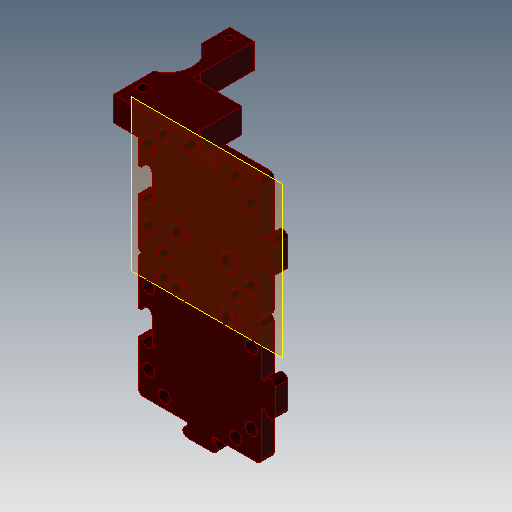
# Autodesk Inventor part: 30_cellSTORM_base
Saved by Autodesk Inventor 2019.4 (Build 234330000, 330)
## iProperties
Created: 2021-07-06
Part Number: 30_cellSTORM_base
Material: Generic
Document SubType Name: Modeling
Designer: diederichbenedict
Density: 1 g/cm^3
Appearance: Smooth - Red
Mass: 29.7217 g
Surface Area: 152.077 cm^2
Volume: 29.7217 cm^3
Author: diederichbenedict
Autodesk Inventor part; units mm, degrees
ref_plane "YZ Plane" through (0, 0, 0) normal (1, 0, 0) x (0, 1, 0)
ref_plane "XZ Plane" through (0, 0, 0) normal (0, 1, 0) x (-1, 0, 0)
ref_plane "XY Plane" through (0, 0, 0) normal (0, 0, 1) x (1, 0, 0)
ref_plane "Work Plane1" through (0, 0, 0) normal (0, 0, 1) x (1, 0, 0)
sketch "Sketch1" plane through (0, 0, 0) normal (0, 0, 1) x (1, 0, 0)
  circle A0 centre (5.7948, 15.4052) radius 2.5 construction
  circle A1 centre (-15.6052, -5.7948) radius 2.5 construction
  line L0 (-20.0856, 39.0762) -> (-20.0856, 40.2052) construction
  line L1 (-20.0856, 40.2052) -> (-38.2052, 40.2052) construction
  arc A2 (-38.2052, 40.2052) -> (-40.2052, 38.2052) centre (-38.2052, 38.2052) ccw construction
  line L2 (-40.2052, 20.2953) -> (-40.2052, 38.2052) construction
  line L3 (-40.2052, 20.2953) -> (-39.0783, 20.2953) construction
  arc A3 (-39.0783, 20.2953) -> (-38.6768, 20.6232) centre (-39.0783, 20.7051) ccw construction
  arc A4 (-34.5391, 20.2052) -> (-38.6768, 20.6232) centre (-36.6291, 20.2052) ccw construction
  line L4 (-34.5391, 20.2052) -> (-34.5391, 10.4067) construction
  arc A5 (-38.647, 9.8643) -> (-34.5391, 10.4067) centre (-36.6023, 10.2052) ccw construction
  line L5 (-38.647, 9.8643) -> (-38.6775, 9.9849) construction
  arc A6 (-38.6775, 9.9849) -> (-39.0762, 10.3249) centre (-39.083, 9.9131) ccw construction
  line L6 (-39.0762, 10.3249) -> (-40.2052, 10.3249) construction
  line L7 (-40.2052, -7.7948) -> (-40.2052, 10.3249) construction
  arc A7 (-40.2052, -7.7948) -> (-38.2052, -9.7948) centre (-38.2052, -7.7948) ccw construction
  line L8 (-38.2052, -9.7948) -> (-20.2052, -9.7948) construction
  line L9 (-20.2052, -9.7948) -> (-20.2052, -10.8453) construction
  arc A8 (-20.6052, -11.3352) -> (-20.2052, -10.8453) centre (-20.7052, -10.8453) ccw construction
  arc A9 (-20.6052, -11.3352) -> (-20.2052, -15.2948) centre (-20.2052, -13.2948) ccw construction
  line L10 (-20.2052, -15.2948) -> (-10.2052, -15.2948) construction
  arc A10 (-10.2052, -15.2948) -> (-9.8052, -11.3352) centre (-10.2052, -13.2948) ccw construction
  arc A11 (-10.2052, -10.8453) -> (-9.8052, -11.3352) centre (-9.7052, -10.8453) ccw construction
  line L11 (-10.2052, -10.8453) -> (-10.2052, -9.7948) construction
  line L12 (-10.2052, -9.7948) -> (7.7948, -9.7948) construction
  arc A12 (7.7948, -9.7948) -> (9.7948, -7.7948) centre (7.7948, -7.7948) ccw construction
  line L13 (9.7948, 10.2052) -> (9.7948, -7.7948) construction
  line L14 (9.7948, 10.2052) -> (10.8453, 10.2052) construction
  arc A13 (11.3352, 9.8052) -> (10.8453, 10.2052) centre (10.8453, 9.7052) ccw construction
  arc A14 (11.3352, 9.8052) -> (15.2948, 10.2052) centre (13.2948, 10.2052) ccw construction
  line L15 (15.2948, 10.2052) -> (15.2948, 20.2052) construction
  arc A15 (15.2948, 20.2052) -> (11.3352, 20.6052) centre (13.2948, 20.2052) ccw construction
  arc A16 (10.8453, 20.2052) -> (11.3352, 20.6052) centre (10.8453, 20.7052) ccw construction
  line L16 (10.8453, 20.2052) -> (9.7948, 20.2052) construction
  line L17 (9.7948, 38.2052) -> (9.7948, 20.2052) construction
  arc A17 (9.7948, 38.2052) -> (7.7948, 40.2052) centre (7.7948, 38.2052) ccw construction
  line L18 (7.7948, 40.2052) -> (-10.1151, 40.2052) construction
  line L19 (-10.1151, 40.2052) -> (-10.1151, 39.0783) construction
  arc A18 (-10.1151, 39.0783) -> (-9.7873, 38.6768) centre (-9.7054, 39.0783) ccw construction
  arc A19 (-10.2052, 34.5391) -> (-9.7873, 38.6768) centre (-10.2052, 36.6291) ccw construction
  line L20 (-10.2052, 34.5391) -> (-20.0038, 34.5391) construction
  arc A20 (-20.5462, 38.647) -> (-20.0038, 34.5391) centre (-20.2052, 36.6023) ccw construction
  line L21 (-20.5462, 38.647) -> (-20.4256, 38.6775) construction
  arc A21 (-20.4256, 38.6775) -> (-20.0856, 39.0762) centre (-20.4974, 39.083) ccw construction
  line L22 (-0.2052, 32.2052) -> (-30.2052, 32.2052) construction
  arc A22 (1.7948, 30.2052) -> (-0.2052, 32.2052) centre (-0.2052, 30.2052) ccw construction
  line L23 (1.7948, 30.2052) -> (1.7948, 0.2052) construction
  arc A23 (-0.2052, -1.7948) -> (1.7948, 0.2052) centre (-0.2052, 0.2052) ccw construction
  line L24 (-0.2052, -1.7948) -> (-30.2052, -1.7948) construction
  arc A24 (-32.2052, 0.2052) -> (-30.2052, -1.7948) centre (-30.2052, 0.2052) ccw construction
  line L25 (-32.2052, 0.2052) -> (-32.2052, 30.2052) construction
  arc A25 (-30.2052, 32.2052) -> (-32.2052, 30.2052) centre (-30.2052, 30.2052) ccw construction
  circle A26 centre (-35.2052, 35.2052) radius 2.425 construction
  circle A27 centre (-29.7052, 36.0052) radius 2.65 construction
  circle A28 centre (-36.0052, 29.7052) radius 2.65 construction
  circle A29 centre (-35.2052, -4.7948) radius 2.425 construction
  circle A30 centre (-29.7052, -5.5948) radius 2.65 construction
  circle A31 centre (-36.0052, 0.7052) radius 2.65 construction
  circle A32 centre (4.7948, 35.2052) radius 2.425 construction
  circle A33 centre (-0.7052, 36.0052) radius 2.65 construction
  circle A34 centre (5.5948, 29.7052) radius 2.65 construction
  circle A35 centre (5.5948, 0.7052) radius 2.65 construction
  circle A36 centre (-0.7052, -5.5948) radius 2.65 construction
  circle A37 centre (4.7948, -4.7948) radius 2.425 construction
  circle A38 centre (5.7948, -34.5948) radius 2.5 construction
  circle A39 centre (-15.6052, -55.7948) radius 2.5 construction
  line L26 (-20.0856, -10.9238) -> (-20.0856, -9.7948) construction
  line L27 (-20.0856, -9.7948) -> (-38.2052, -9.7948) construction
  arc A40 (-38.2052, -9.7948) -> (-40.2052, -11.7948) centre (-38.2052, -11.7948) ccw construction
  line L28 (-40.2052, -29.7047) -> (-40.2052, -11.7948) construction
  line L29 (-40.2052, -29.7047) -> (-39.0783, -29.7047) construction
  arc A41 (-39.0783, -29.7047) -> (-38.6768, -29.3768) centre (-39.0783, -29.2949) ccw construction
  arc A42 (-34.5391, -29.7948) -> (-38.6768, -29.3768) centre (-36.6291, -29.7948) ccw construction
  line L30 (-34.5391, -29.7948) -> (-34.5391, -39.5933) construction
  arc A43 (-38.647, -40.1357) -> (-34.5391, -39.5933) centre (-36.6023, -39.7948) ccw construction
  line L31 (-38.647, -40.1357) -> (-38.6775, -40.0151) construction
  arc A44 (-38.6775, -40.0151) -> (-39.0762, -39.6751) centre (-39.083, -40.0869) ccw construction
  line L32 (-39.0762, -39.6751) -> (-40.2052, -39.6751) construction
  line L33 (-40.2052, -57.7948) -> (-40.2052, -39.6751) construction
  arc A45 (-40.2052, -57.7948) -> (-38.2052, -59.7948) centre (-38.2052, -57.7948) ccw construction
  line L34 (-38.2052, -59.7948) -> (-20.2052, -59.7948) construction
  line L35 (-20.2052, -59.7948) -> (-20.2052, -60.8453) construction
  arc A46 (-20.6052, -61.3352) -> (-20.2052, -60.8453) centre (-20.7052, -60.8453) ccw construction
  arc A47 (-20.6052, -61.3352) -> (-20.2052, -65.2948) centre (-20.2052, -63.2948) ccw construction
  line L36 (-20.2052, -65.2948) -> (-10.2052, -65.2948) construction
  arc A48 (-10.2052, -65.2948) -> (-9.8052, -61.3352) centre (-10.2052, -63.2948) ccw construction
  arc A49 (-10.2052, -60.8453) -> (-9.8052, -61.3352) centre (-9.7052, -60.8453) ccw construction
  line L37 (-10.2052, -60.8453) -> (-10.2052, -59.7948) construction
  line L38 (-10.2052, -59.7948) -> (7.7948, -59.7948) construction
  arc A50 (7.7948, -59.7948) -> (9.7948, -57.7948) centre (7.7948, -57.7948) ccw construction
  line L39 (9.7948, -39.7948) -> (9.7948, -57.7948) construction
  line L40 (9.7948, -39.7948) -> (10.8453, -39.7948) construction
  arc A51 (11.3352, -40.1948) -> (10.8453, -39.7948) centre (10.8453, -40.2948) ccw construction
  arc A52 (11.3352, -40.1948) -> (15.2948, -39.7948) centre (13.2948, -39.7948) ccw construction
  line L41 (15.2948, -39.7948) -> (15.2948, -29.7948) construction
  arc A53 (15.2948, -29.7948) -> (11.3352, -29.3948) centre (13.2948, -29.7948) ccw construction
  arc A54 (10.8453, -29.7948) -> (11.3352, -29.3948) centre (10.8453, -29.2948) ccw construction
  line L42 (10.8453, -29.7948) -> (9.7948, -29.7948) construction
  line L43 (9.7948, -11.7948) -> (9.7948, -29.7948) construction
  arc A55 (9.7948, -11.7948) -> (7.7948, -9.7948) centre (7.7948, -11.7948) ccw construction
  line L44 (7.7948, -9.7948) -> (-10.1151, -9.7948) construction
  line L45 (-10.1151, -9.7948) -> (-10.1151, -10.9217) construction
  arc A56 (-10.1151, -10.9217) -> (-9.7873, -11.3232) centre (-9.7054, -10.9217) ccw construction
  arc A57 (-10.2052, -15.4609) -> (-9.7873, -11.3232) centre (-10.2052, -13.3709) ccw construction
  line L46 (-10.2052, -15.4609) -> (-20.0038, -15.4609) construction
  arc A58 (-20.5462, -11.353) -> (-20.0038, -15.4609) centre (-20.2052, -13.3977) ccw construction
  line L47 (-20.5462, -11.353) -> (-20.4256, -11.3225) construction
  arc A59 (-20.4256, -11.3225) -> (-20.0856, -10.9238) centre (-20.4974, -10.917) ccw construction
  line L48 (-0.2052, -17.7948) -> (-30.2052, -17.7948) construction
  arc A60 (1.7948, -19.7948) -> (-0.2052, -17.7948) centre (-0.2052, -19.7948) ccw construction
  line L49 (1.7948, -19.7948) -> (1.7948, -49.7948) construction
  arc A61 (-0.2052, -51.7948) -> (1.7948, -49.7948) centre (-0.2052, -49.7948) ccw construction
  line L50 (-0.2052, -51.7948) -> (-30.2052, -51.7948) construction
  arc A62 (-32.2052, -49.7948) -> (-30.2052, -51.7948) centre (-30.2052, -49.7948) ccw construction
  line L51 (-32.2052, -49.7948) -> (-32.2052, -19.7948) construction
  arc A63 (-30.2052, -17.7948) -> (-32.2052, -19.7948) centre (-30.2052, -19.7948) ccw construction
  circle A64 centre (-35.2052, -14.7948) radius 2.425 construction
  circle A65 centre (-29.7052, -13.9948) radius 2.65 construction
  circle A66 centre (-36.0052, -20.2948) radius 2.65 construction
  circle A67 centre (-35.2052, -54.7948) radius 2.425 construction
  circle A68 centre (-29.7052, -55.5948) radius 2.65 construction
  circle A69 centre (-36.0052, -49.2948) radius 2.65 construction
  circle A70 centre (4.7948, -14.7948) radius 2.425 construction
  circle A71 centre (-0.7052, -13.9948) radius 2.65 construction
  circle A72 centre (5.5948, -20.2948) radius 2.65 construction
  circle A73 centre (5.5948, -49.2948) radius 2.65 construction
  circle A74 centre (-0.7052, -55.5948) radius 2.65 construction
  circle A75 centre (4.7948, -54.7948) radius 2.425 construction
  circle A76 centre (5.7948, 15.4052) radius 2.5 projected
  circle A77 centre (-15.6052, -5.7948) radius 2.5 projected
  line L52 (-20.0856, 39.0762) -> (-20.0856, 40.2052) projected
  line L53 (-20.0856, 40.2052) -> (-38.2052, 40.2052) projected
  arc A78 (-38.2052, 40.2052) -> (-40.2052, 38.2052) centre (-38.2052, 38.2052) ccw projected
  line L54 (-40.2052, 20.2953) -> (-40.2052, 38.2052) projected
  line L55 (-40.2052, 20.2953) -> (-39.0783, 20.2953) projected
  arc A79 (-39.0783, 20.2953) -> (-38.6768, 20.6232) centre (-39.0783, 20.7051) ccw projected
  arc A80 (-34.5391, 20.2052) -> (-38.6768, 20.6232) centre (-36.6291, 20.2052) ccw projected
  line L56 (-34.5391, 20.2052) -> (-34.5391, 10.4067) projected
  arc A81 (-38.647, 9.8643) -> (-34.5391, 10.4067) centre (-36.6023, 10.2052) ccw projected
  line L57 (-38.647, 9.8643) -> (-38.6775, 9.9849) projected
  arc A82 (-38.6775, 9.9849) -> (-39.0762, 10.3249) centre (-39.083, 9.9131) ccw projected
  line L58 (-39.0762, 10.3249) -> (-40.2052, 10.3249) projected
  line L59 (-40.2052, -7.7948) -> (-40.2052, 10.3249) projected
  arc A83 (-40.2052, -7.7948) -> (-38.2052, -9.7948) centre (-38.2052, -7.7948) ccw projected
  line L60 (-38.2052, -9.7948) -> (-20.2052, -9.7948) projected
  line L61 (-20.2052, -9.7948) -> (-20.2052, -10.8453) projected
  arc A84 (-20.6052, -11.3352) -> (-20.2052, -10.8453) centre (-20.7052, -10.8453) ccw projected
  arc A85 (-20.6052, -11.3352) -> (-20.2052, -15.2948) centre (-20.2052, -13.2948) ccw projected
  line L62 (-20.2052, -15.2948) -> (-10.2052, -15.2948) projected
  arc A86 (-10.2052, -15.2948) -> (-9.8052, -11.3352) centre (-10.2052, -13.2948) ccw projected
  arc A87 (-10.2052, -10.8453) -> (-9.8052, -11.3352) centre (-9.7052, -10.8453) ccw projected
  line L63 (-10.2052, -10.8453) -> (-10.2052, -9.7948) projected
  line L64 (-10.2052, -9.7948) -> (7.7948, -9.7948) projected
  arc A88 (7.7948, -9.7948) -> (9.7948, -7.7948) centre (7.7948, -7.7948) ccw projected
  line L65 (9.7948, 10.2052) -> (9.7948, -7.7948) projected
  line L66 (9.7948, 10.2052) -> (10.8453, 10.2052) projected
  arc A89 (11.3352, 9.8052) -> (10.8453, 10.2052) centre (10.8453, 9.7052) ccw projected
  arc A90 (11.3352, 9.8052) -> (15.2948, 10.2052) centre (13.2948, 10.2052) ccw projected
  line L67 (15.2948, 10.2052) -> (15.2948, 20.2052) projected
  arc A91 (15.2948, 20.2052) -> (11.3352, 20.6052) centre (13.2948, 20.2052) ccw projected
  arc A92 (10.8453, 20.2052) -> (11.3352, 20.6052) centre (10.8453, 20.7052) ccw projected
  line L68 (10.8453, 20.2052) -> (9.7948, 20.2052) projected
  line L69 (9.7948, 38.2052) -> (9.7948, 20.2052) projected
  arc A93 (9.7948, 38.2052) -> (7.7948, 40.2052) centre (7.7948, 38.2052) ccw projected
  line L70 (7.7948, 40.2052) -> (-10.1151, 40.2052) projected
  line L71 (-10.1151, 40.2052) -> (-10.1151, 39.0783) projected
  arc A94 (-10.1151, 39.0783) -> (-9.7873, 38.6768) centre (-9.7054, 39.0783) ccw projected
  arc A95 (-10.2052, 34.5391) -> (-9.7873, 38.6768) centre (-10.2052, 36.6291) ccw projected
  line L72 (-10.2052, 34.5391) -> (-20.0038, 34.5391) projected
  arc A96 (-20.5462, 38.647) -> (-20.0038, 34.5391) centre (-20.2052, 36.6023) ccw projected
  line L73 (-20.5462, 38.647) -> (-20.4256, 38.6775) projected
  arc A97 (-20.4256, 38.6775) -> (-20.0856, 39.0762) centre (-20.4974, 39.083) ccw projected
  line L74 (-0.2052, 32.2052) -> (-30.2052, 32.2052) projected
  arc A98 (1.7948, 30.2052) -> (-0.2052, 32.2052) centre (-0.2052, 30.2052) ccw projected
  line L75 (1.7948, 30.2052) -> (1.7948, 0.2052) projected
  arc A99 (-0.2052, -1.7948) -> (1.7948, 0.2052) centre (-0.2052, 0.2052) ccw projected
  line L76 (-0.2052, -1.7948) -> (-30.2052, -1.7948) projected
  arc A100 (-32.2052, 0.2052) -> (-30.2052, -1.7948) centre (-30.2052, 0.2052) ccw projected
  line L77 (-32.2052, 0.2052) -> (-32.2052, 30.2052) projected
  arc A101 (-30.2052, 32.2052) -> (-32.2052, 30.2052) centre (-30.2052, 30.2052) ccw projected
  circle A102 centre (-35.2052, 35.2052) radius 2.425 projected
  circle A103 centre (-29.7052, 36.0052) radius 2.65 projected
  circle A104 centre (-36.0052, 29.7052) radius 2.65 projected
  circle A105 centre (-35.2052, -4.7948) radius 2.425 projected
  circle A106 centre (-29.7052, -5.5948) radius 2.65 projected
  circle A107 centre (-36.0052, 0.7052) radius 2.65 projected
  circle A108 centre (4.7948, 35.2052) radius 2.425 projected
  circle A109 centre (-0.7052, 36.0052) radius 2.65 projected
  circle A110 centre (5.5948, 29.7052) radius 2.65 projected
  circle A111 centre (5.5948, 0.7052) radius 2.65 projected
  circle A112 centre (-0.7052, -5.5948) radius 2.65 projected
  circle A113 centre (4.7948, -4.7948) radius 2.425 projected
  circle A114 centre (5.7948, -34.5948) radius 2.5 projected
  circle A115 centre (-15.6052, -55.7948) radius 2.5 projected
  line L78 (-20.0856, -10.9238) -> (-20.0856, -9.7948) projected
  line L79 (-20.0856, -9.7948) -> (-38.2052, -9.7948) projected
  arc A116 (-38.2052, -9.7948) -> (-40.2052, -11.7948) centre (-38.2052, -11.7948) ccw projected
  line L80 (-40.2052, -29.7047) -> (-40.2052, -11.7948) projected
  line L81 (-40.2052, -29.7047) -> (-39.0783, -29.7047) projected
  arc A117 (-39.0783, -29.7047) -> (-38.6768, -29.3768) centre (-39.0783, -29.2949) ccw projected
  arc A118 (-34.5391, -29.7948) -> (-38.6768, -29.3768) centre (-36.6291, -29.7948) ccw projected
  line L82 (-34.5391, -29.7948) -> (-34.5391, -39.5933) projected
  arc A119 (-38.647, -40.1357) -> (-34.5391, -39.5933) centre (-36.6023, -39.7948) ccw projected
  line L83 (-38.647, -40.1357) -> (-38.6775, -40.0151) projected
  arc A120 (-38.6775, -40.0151) -> (-39.0762, -39.6751) centre (-39.083, -40.0869) ccw projected
  line L84 (-39.0762, -39.6751) -> (-40.2052, -39.6751) projected
  line L85 (-40.2052, -57.7948) -> (-40.2052, -39.6751) projected
  arc A121 (-40.2052, -57.7948) -> (-38.2052, -59.7948) centre (-38.2052, -57.7948) ccw projected
  line L86 (-38.2052, -59.7948) -> (-20.2052, -59.7948) projected
  line L87 (-20.2052, -59.7948) -> (-20.2052, -60.8453) projected
  arc A122 (-20.6052, -61.3352) -> (-20.2052, -60.8453) centre (-20.7052, -60.8453) ccw projected
  arc A123 (-20.6052, -61.3352) -> (-20.2052, -65.2948) centre (-20.2052, -63.2948) ccw projected
  line L88 (-20.2052, -65.2948) -> (-10.2052, -65.2948) projected
  arc A124 (-10.2052, -65.2948) -> (-9.8052, -61.3352) centre (-10.2052, -63.2948) ccw projected
  arc A125 (-10.2052, -60.8453) -> (-9.8052, -61.3352) centre (-9.7052, -60.8453) ccw projected
  line L89 (-10.2052, -60.8453) -> (-10.2052, -59.7948) projected
  line L90 (-10.2052, -59.7948) -> (7.7948, -59.7948) projected
  arc A126 (7.7948, -59.7948) -> (9.7948, -57.7948) centre (7.7948, -57.7948) ccw projected
  line L91 (9.7948, -39.7948) -> (9.7948, -57.7948) projected
  line L92 (9.7948, -39.7948) -> (10.8453, -39.7948) projected
  arc A127 (11.3352, -40.1948) -> (10.8453, -39.7948) centre (10.8453, -40.2948) ccw projected
  arc A128 (11.3352, -40.1948) -> (15.2948, -39.7948) centre (13.2948, -39.7948) ccw projected
  line L93 (15.2948, -39.7948) -> (15.2948, -29.7948) projected
  arc A129 (15.2948, -29.7948) -> (11.3352, -29.3948) centre (13.2948, -29.7948) ccw projected
  arc A130 (10.8453, -29.7948) -> (11.3352, -29.3948) centre (10.8453, -29.2948) ccw projected
  line L94 (10.8453, -29.7948) -> (9.7948, -29.7948) projected
  line L95 (9.7948, -11.7948) -> (9.7948, -29.7948) projected
  arc A131 (9.7948, -11.7948) -> (7.7948, -9.7948) centre (7.7948, -11.7948) ccw projected
  line L96 (7.7948, -9.7948) -> (-10.1151, -9.7948) projected
  line L97 (-10.1151, -9.7948) -> (-10.1151, -10.9217) projected
  arc A132 (-10.1151, -10.9217) -> (-9.7873, -11.3232) centre (-9.7054, -10.9217) ccw projected
  arc A133 (-10.2052, -15.4609) -> (-9.7873, -11.3232) centre (-10.2052, -13.3709) ccw projected
  line L98 (-10.2052, -15.4609) -> (-20.0038, -15.4609) projected
  arc A134 (-20.5462, -11.353) -> (-20.0038, -15.4609) centre (-20.2052, -13.3977) ccw projected
  line L99 (-20.5462, -11.353) -> (-20.4256, -11.3225) projected
  arc A135 (-20.4256, -11.3225) -> (-20.0856, -10.9238) centre (-20.4974, -10.917) ccw projected
  line L100 (-0.2052, -17.7948) -> (-30.2052, -17.7948) projected
  arc A136 (1.7948, -19.7948) -> (-0.2052, -17.7948) centre (-0.2052, -19.7948) ccw projected
  line L101 (1.7948, -19.7948) -> (1.7948, -49.7948) projected
  arc A137 (-0.2052, -51.7948) -> (1.7948, -49.7948) centre (-0.2052, -49.7948) ccw projected
  line L102 (-0.2052, -51.7948) -> (-30.2052, -51.7948) projected
  arc A138 (-32.2052, -49.7948) -> (-30.2052, -51.7948) centre (-30.2052, -49.7948) ccw projected
  line L103 (-32.2052, -49.7948) -> (-32.2052, -19.7948) projected
  arc A139 (-30.2052, -17.7948) -> (-32.2052, -19.7948) centre (-30.2052, -19.7948) ccw projected
  circle A140 centre (-35.2052, -14.7948) radius 2.425 projected
  circle A141 centre (-29.7052, -13.9948) radius 2.65 projected
  circle A142 centre (-36.0052, -20.2948) radius 2.65 projected
  circle A143 centre (-35.2052, -54.7948) radius 2.425 projected
  circle A144 centre (-29.7052, -55.5948) radius 2.65 projected
  circle A145 centre (-36.0052, -49.2948) radius 2.65 projected
  circle A146 centre (4.7948, -14.7948) radius 2.425 projected
  circle A147 centre (-0.7052, -13.9948) radius 2.65 projected
  circle A148 centre (5.5948, -20.2948) radius 2.65 projected
  circle A149 centre (5.5948, -49.2948) radius 2.65 projected
  circle A150 centre (-0.7052, -55.5948) radius 2.65 projected
  circle A151 centre (4.7948, -54.7948) radius 2.425 projected
  point P0 (0, 0)
extrude "Extrusion1" add sketch "Sketch1" against normal blind 5 contours A76 | A77 | A97 L73 A96 L72 A95 A94 L71 L70 A93 L69 L68 A92 A91 L67 A90 A89 L66 L65 A88 L64 L63 A87 A86 L62 A85 A134 L99 A135 L78 L79 L60 A83 L59 L58 A82 L57 A81 L56 A80 A79 L55 L54 A78 L53 L52 | L60 L61 A84 A85 A134 L98 A133 A132 L97 L64 A131 L95 L94 A130 A129 L93 A128 A127 L92 L91 A126 L90 L89 A125 A124 L88 A123 A122 L87 L86 A121 L85 L84 A120 L83 A119 L82 A118 A117 L81 L80 A116 | L79 L78 A135 L99 A134 A85 A84 L61 | A85 L62 A86 A87 L63 L64 L97 A132 A133 L98 A134 | A98 L75 A99 L76 A100 L77 A101 L74 | A102 | A103 | A104 | A105 | A106 | A107 | A108 | A109 | A110 | A111 | A112 | A113 | A114 | A115 | A136 L101 A137 L102 A138 L103 A139 L100 | A140 | A141 | A142 | A143 | A144 | A145 | A146 | A147 | A148 | A149 | A150 | A151
sketch "Sketch2" plane through (0, 0, 0) normal (0, 0, 1) x (-1, 0, 0)
  circle A0 centre (23.4848, -4.9552) radius 1.5 projected
  circle A1 centre (23.4848, 15.0448) radius 1.25 projected
  circle A2 centre (3.4848, -4.9552) radius 1.25 projected
  circle A3 centre (3.4848, 15.0448) radius 1.5 projected
  point P0 (0, 0)
hole "Hole1" at (-23.4848, -15.0448, 0) at (-23.4848, 4.9552, 0) at (-3.4848, 4.9552, 0) at (-3.4848, -15.0448, 0) direction (0, 0, -1) diameter 2.9 end through all counterbore diameter 7 counterbore depth 3
sketch "Sketch3" plane through (0, 0, -5) normal (0, 0, -1) x (-1, 0, 0)
  circle A0 centre (-5.5948, -49.2948) radius 2.65 construction
  circle A1 centre (3.4848, 4.9552) radius 1.45 construction
  circle A2 centre (23.4848, -15.0448) radius 1.45 construction
  circle A3 centre (23.4848, 4.9552) radius 1.45 construction
  circle A4 centre (3.4848, -15.0448) radius 1.45 construction
  arc A5 (20.0856, 39.0762) -> (20.4256, 38.6775) centre (20.4974, 39.083) ccw construction
  line L0 (20.4256, 38.6775) -> (20.5462, 38.647) construction
  arc A6 (20.0038, 34.5391) -> (20.5462, 38.647) centre (20.2052, 36.6023) ccw construction
  line L1 (20.0038, 34.5391) -> (10.2052, 34.5391) construction
  arc A7 (9.7873, 38.6768) -> (10.2052, 34.5391) centre (10.2052, 36.6291) ccw construction
  arc A8 (9.7873, 38.6768) -> (10.1151, 39.0783) centre (9.7054, 39.0783) ccw construction
  line L2 (10.1151, 39.0783) -> (10.1151, 40.2052) construction
  line L3 (10.1151, 40.2052) -> (-7.7948, 40.2052) construction
  arc A9 (-7.7948, 40.2052) -> (-9.7948, 38.2052) centre (-7.7948, 38.2052) ccw construction
  line L4 (-9.7948, 38.2052) -> (-9.7948, 20.2052) construction
  line L5 (-9.7948, 20.2052) -> (-10.8453, 20.2052) construction
  arc A10 (-11.3352, 20.6052) -> (-10.8453, 20.2052) centre (-10.8453, 20.7052) ccw construction
  arc A11 (-11.3352, 20.6052) -> (-15.2948, 20.2052) centre (-13.2948, 20.2052) ccw construction
  line L6 (-15.2948, 20.2052) -> (-15.2948, 10.2052) construction
  arc A12 (-15.2948, 10.2052) -> (-11.3352, 9.8052) centre (-13.2948, 10.2052) ccw construction
  arc A13 (-10.8453, 10.2052) -> (-11.3352, 9.8052) centre (-10.8453, 9.7052) ccw construction
  line L7 (-10.8453, 10.2052) -> (-9.7948, 10.2052) construction
  line L8 (-9.7948, 10.2052) -> (-9.7948, -7.7948) construction
  arc A14 (-9.7948, -7.7948) -> (-7.7948, -9.7948) centre (-7.7948, -7.7948) ccw construction
  arc A15 (-7.7948, -9.7948) -> (-9.7948, -11.7948) centre (-7.7948, -11.7948) ccw construction
  line L9 (-9.7948, -11.7948) -> (-9.7948, -29.7948) construction
  line L10 (-9.7948, -29.7948) -> (-10.8453, -29.7948) construction
  arc A16 (-11.3352, -29.3948) -> (-10.8453, -29.7948) centre (-10.8453, -29.2948) ccw construction
  arc A17 (-11.3352, -29.3948) -> (-15.2948, -29.7948) centre (-13.2948, -29.7948) ccw construction
  line L11 (-15.2948, -29.7948) -> (-15.2948, -39.7948) construction
  arc A18 (-15.2948, -39.7948) -> (-11.3352, -40.1948) centre (-13.2948, -39.7948) ccw construction
  arc A19 (-10.8453, -39.7948) -> (-11.3352, -40.1948) centre (-10.8453, -40.2948) ccw construction
  line L12 (-10.8453, -39.7948) -> (-9.7948, -39.7948) construction
  line L13 (-9.7948, -39.7948) -> (-9.7948, -57.7948) construction
  arc A20 (-9.7948, -57.7948) -> (-7.7948, -59.7948) centre (-7.7948, -57.7948) ccw construction
  line L14 (-7.7948, -59.7948) -> (10.2052, -59.7948) construction
  line L15 (10.2052, -59.7948) -> (10.2052, -60.8453) construction
  arc A21 (9.8052, -61.3352) -> (10.2052, -60.8453) centre (9.7052, -60.8453) ccw construction
  arc A22 (9.8052, -61.3352) -> (10.2052, -65.2948) centre (10.2052, -63.2948) ccw construction
  line L16 (10.2052, -65.2948) -> (20.2052, -65.2948) construction
  arc A23 (20.2052, -65.2948) -> (20.6052, -61.3352) centre (20.2052, -63.2948) ccw construction
  arc A24 (20.2052, -60.8453) -> (20.6052, -61.3352) centre (20.7052, -60.8453) ccw construction
  line L17 (20.2052, -60.8453) -> (20.2052, -59.7948) construction
  line L18 (20.2052, -59.7948) -> (38.2052, -59.7948) construction
  arc A25 (38.2052, -59.7948) -> (40.2052, -57.7948) centre (38.2052, -57.7948) ccw construction
  line L19 (40.2052, -57.7948) -> (40.2052, -39.6751) construction
  line L20 (40.2052, -39.6751) -> (39.0762, -39.6751) construction
  arc A26 (39.0762, -39.6751) -> (38.6775, -40.0151) centre (39.083, -40.0869) ccw construction
  line L21 (38.6775, -40.0151) -> (38.647, -40.1357) construction
  arc A27 (34.5391, -39.5933) -> (38.647, -40.1357) centre (36.6023, -39.7948) ccw construction
  line L22 (34.5391, -39.5933) -> (34.5391, -29.7948) construction
  arc A28 (38.6768, -29.3768) -> (34.5391, -29.7948) centre (36.6291, -29.7948) ccw construction
  arc A29 (38.6768, -29.3768) -> (39.0783, -29.7047) centre (39.0783, -29.2949) ccw construction
  line L23 (39.0783, -29.7047) -> (40.2052, -29.7047) construction
  line L24 (40.2052, -29.7047) -> (40.2052, -11.7948) construction
  arc A30 (40.2052, -11.7948) -> (38.2052, -9.7948) centre (38.2052, -11.7948) ccw construction
  arc A31 (38.2052, -9.7948) -> (40.2052, -7.7948) centre (38.2052, -7.7948) ccw construction
  line L25 (40.2052, -7.7948) -> (40.2052, 10.3249) construction
  line L26 (40.2052, 10.3249) -> (39.0762, 10.3249) construction
  arc A32 (39.0762, 10.3249) -> (38.6775, 9.9849) centre (39.083, 9.9131) ccw construction
  line L27 (38.6775, 9.9849) -> (38.647, 9.8643) construction
  arc A33 (34.5391, 10.4067) -> (38.647, 9.8643) centre (36.6023, 10.2052) ccw construction
  line L28 (34.5391, 10.4067) -> (34.5391, 20.2052) construction
  arc A34 (38.6768, 20.6232) -> (34.5391, 20.2052) centre (36.6291, 20.2052) ccw construction
  arc A35 (38.6768, 20.6232) -> (39.0783, 20.2953) centre (39.0783, 20.7051) ccw construction
  line L29 (39.0783, 20.2953) -> (40.2052, 20.2953) construction
  line L30 (40.2052, 20.2953) -> (40.2052, 38.2052) construction
  arc A36 (40.2052, 38.2052) -> (38.2052, 40.2052) centre (38.2052, 38.2052) ccw construction
  line L31 (38.2052, 40.2052) -> (20.0856, 40.2052) construction
  line L32 (20.0856, 40.2052) -> (20.0856, 39.0762) construction
  line L33 (-9.4152, -56.1947) -> (33.5832, -56.1947) construction
  circle A37 centre (-5.7948, -34.5948) radius 2.5 construction
  circle A38 centre (15.6052, -55.7948) radius 2.5 construction
  line L34 (20.0856, -10.9238) -> (20.0856, -9.7948) construction
  line L35 (20.0856, -9.7948) -> (38.2052, -9.7948) construction
  arc A39 (40.2052, -11.7948) -> (38.2052, -9.7948) centre (38.2052, -11.7948) ccw construction
  line L36 (40.2052, -29.7047) -> (40.2052, -11.7948) construction
  line L37 (40.2052, -29.7047) -> (39.0783, -29.7047) construction
  arc A40 (38.6768, -29.3768) -> (39.0783, -29.7047) centre (39.0783, -29.2949) ccw construction
  arc A41 (38.6768, -29.3768) -> (34.5391, -29.7948) centre (36.6291, -29.7948) ccw construction
  line L38 (34.5391, -29.7948) -> (34.5391, -39.5933) construction
  arc A42 (34.5391, -39.5933) -> (38.647, -40.1357) centre (36.6023, -39.7948) ccw construction
  line L39 (38.647, -40.1357) -> (38.6775, -40.0151) construction
  arc A43 (39.0762, -39.6751) -> (38.6775, -40.0151) centre (39.083, -40.0869) ccw construction
  line L40 (39.0762, -39.6751) -> (40.2052, -39.6751) construction
  line L41 (40.2052, -57.7948) -> (40.2052, -39.6751) construction
  arc A44 (38.2052, -59.7948) -> (40.2052, -57.7948) centre (38.2052, -57.7948) ccw construction
  line L42 (38.2052, -59.7948) -> (20.2052, -59.7948) construction
  line L43 (20.2052, -59.7948) -> (20.2052, -60.8453) construction
  arc A45 (20.2052, -60.8453) -> (20.6052, -61.3352) centre (20.7052, -60.8453) ccw construction
  arc A46 (20.2052, -65.2948) -> (20.6052, -61.3352) centre (20.2052, -63.2948) ccw construction
  line L44 (20.2052, -65.2948) -> (10.2052, -65.2948) construction
  arc A47 (9.8052, -61.3352) -> (10.2052, -65.2948) centre (10.2052, -63.2948) ccw construction
  arc A48 (9.8052, -61.3352) -> (10.2052, -60.8453) centre (9.7052, -60.8453) ccw construction
  line L45 (10.2052, -60.8453) -> (10.2052, -59.7948) construction
  line L46 (10.2052, -59.7948) -> (-7.7948, -59.7948) construction
  arc A49 (-9.7948, -57.7948) -> (-7.7948, -59.7948) centre (-7.7948, -57.7948) ccw construction
  line L47 (-9.7948, -39.7948) -> (-9.7948, -57.7948) construction
  line L48 (-9.7948, -39.7948) -> (-10.8453, -39.7948) construction
  arc A50 (-10.8453, -39.7948) -> (-11.3352, -40.1948) centre (-10.8453, -40.2948) ccw construction
  arc A51 (-15.2948, -39.7948) -> (-11.3352, -40.1948) centre (-13.2948, -39.7948) ccw construction
  line L49 (-15.2948, -39.7948) -> (-15.2948, -29.7948) construction
  arc A52 (-11.3352, -29.3948) -> (-15.2948, -29.7948) centre (-13.2948, -29.7948) ccw construction
  arc A53 (-11.3352, -29.3948) -> (-10.8453, -29.7948) centre (-10.8453, -29.2948) ccw construction
  line L50 (-10.8453, -29.7948) -> (-9.7948, -29.7948) construction
  line L51 (-9.7948, -11.7948) -> (-9.7948, -29.7948) construction
  arc A54 (-7.7948, -9.7948) -> (-9.7948, -11.7948) centre (-7.7948, -11.7948) ccw construction
  line L52 (-7.7948, -9.7948) -> (10.1151, -9.7948) construction
  line L53 (10.1151, -9.7948) -> (10.1151, -10.9217) construction
  arc A55 (9.7873, -11.3232) -> (10.1151, -10.9217) centre (9.7054, -10.9217) ccw construction
  arc A56 (9.7873, -11.3232) -> (10.2052, -15.4609) centre (10.2052, -13.3709) ccw construction
  line L54 (10.2052, -15.4609) -> (20.0038, -15.4609) construction
  arc A57 (20.0038, -15.4609) -> (20.5462, -11.353) centre (20.2052, -13.3977) ccw construction
  line L55 (20.5462, -11.353) -> (20.4256, -11.3225) construction
  arc A58 (20.0856, -10.9238) -> (20.4256, -11.3225) centre (20.4974, -10.917) ccw construction
  line L56 (0.2052, -17.7948) -> (30.2052, -17.7948) construction
  arc A59 (0.2052, -17.7948) -> (-1.7948, -19.7948) centre (0.2052, -19.7948) ccw construction
  line L57 (-1.7948, -19.7948) -> (-1.7948, -49.7948) construction
  arc A60 (-1.7948, -49.7948) -> (0.2052, -51.7948) centre (0.2052, -49.7948) ccw construction
  line L58 (0.2052, -51.7948) -> (30.2052, -51.7948) construction
  arc A61 (30.2052, -51.7948) -> (32.2052, -49.7948) centre (30.2052, -49.7948) ccw construction
  line L59 (32.2052, -49.7948) -> (32.2052, -19.7948) construction
  arc A62 (32.2052, -19.7948) -> (30.2052, -17.7948) centre (30.2052, -19.7948) ccw construction
  circle A63 centre (35.2052, -14.7948) radius 2.425 construction
  circle A64 centre (29.7052, -13.9948) radius 2.65 construction
  circle A65 centre (36.0052, -20.2948) radius 2.65 construction
  circle A66 centre (35.2052, -54.7948) radius 2.425 construction
  circle A67 centre (29.7052, -55.5948) radius 2.65 construction
  circle A68 centre (36.0052, -49.2948) radius 2.65 construction
  circle A69 centre (-4.7948, -14.7948) radius 2.425 construction
  circle A70 centre (0.7052, -13.9948) radius 2.65 construction
  circle A71 centre (-5.5948, -20.2948) radius 2.65 construction
  circle A72 centre (-5.5948, -49.2948) radius 2.65 construction
  circle A73 centre (0.7052, -55.5948) radius 2.65 construction
  circle A74 centre (-4.7948, -54.7948) radius 2.425 construction
  circle A75 centre (-5.7948, 15.4052) radius 2.5 construction
  circle A76 centre (15.6052, -5.7948) radius 2.5 construction
  line L60 (20.0856, 39.0762) -> (20.0856, 40.2052) construction
  line L61 (20.0856, 40.2052) -> (38.2052, 40.2052) construction
  arc A77 (40.2052, 38.2052) -> (38.2052, 40.2052) centre (38.2052, 38.2052) ccw construction
  line L62 (40.2052, 20.2953) -> (40.2052, 38.2052) construction
  line L63 (40.2052, 20.2953) -> (39.0783, 20.2953) construction
  arc A78 (38.6768, 20.6232) -> (39.0783, 20.2953) centre (39.0783, 20.7051) ccw construction
  arc A79 (38.6768, 20.6232) -> (34.5391, 20.2052) centre (36.6291, 20.2052) ccw construction
  line L64 (34.5391, 20.2052) -> (34.5391, 10.4067) construction
  arc A80 (34.5391, 10.4067) -> (38.647, 9.8643) centre (36.6023, 10.2052) ccw construction
  line L65 (38.647, 9.8643) -> (38.6775, 9.9849) construction
  arc A81 (39.0762, 10.3249) -> (38.6775, 9.9849) centre (39.083, 9.9131) ccw construction
  line L66 (39.0762, 10.3249) -> (40.2052, 10.3249) construction
  line L67 (40.2052, -7.7948) -> (40.2052, 10.3249) construction
  arc A82 (38.2052, -9.7948) -> (40.2052, -7.7948) centre (38.2052, -7.7948) ccw construction
  line L68 (38.2052, -9.7948) -> (20.2052, -9.7948) construction
  line L69 (20.2052, -9.7948) -> (20.2052, -10.8453) construction
  arc A83 (20.2052, -10.8453) -> (20.6052, -11.3352) centre (20.7052, -10.8453) ccw construction
  arc A84 (20.2052, -15.2948) -> (20.6052, -11.3352) centre (20.2052, -13.2948) ccw construction
  line L70 (20.2052, -15.2948) -> (10.2052, -15.2948) construction
  arc A85 (9.8052, -11.3352) -> (10.2052, -15.2948) centre (10.2052, -13.2948) ccw construction
  arc A86 (9.8052, -11.3352) -> (10.2052, -10.8453) centre (9.7052, -10.8453) ccw construction
  line L71 (10.2052, -10.8453) -> (10.2052, -9.7948) construction
  line L72 (10.2052, -9.7948) -> (-7.7948, -9.7948) construction
  arc A87 (-9.7948, -7.7948) -> (-7.7948, -9.7948) centre (-7.7948, -7.7948) ccw construction
  line L73 (-9.7948, 10.2052) -> (-9.7948, -7.7948) construction
  line L74 (-9.7948, 10.2052) -> (-10.8453, 10.2052) construction
  arc A88 (-10.8453, 10.2052) -> (-11.3352, 9.8052) centre (-10.8453, 9.7052) ccw construction
  arc A89 (-15.2948, 10.2052) -> (-11.3352, 9.8052) centre (-13.2948, 10.2052) ccw construction
  line L75 (-15.2948, 10.2052) -> (-15.2948, 20.2052) construction
  arc A90 (-11.3352, 20.6052) -> (-15.2948, 20.2052) centre (-13.2948, 20.2052) ccw construction
  arc A91 (-11.3352, 20.6052) -> (-10.8453, 20.2052) centre (-10.8453, 20.7052) ccw construction
  line L76 (-10.8453, 20.2052) -> (-9.7948, 20.2052) construction
  line L77 (-9.7948, 38.2052) -> (-9.7948, 20.2052) construction
  arc A92 (-7.7948, 40.2052) -> (-9.7948, 38.2052) centre (-7.7948, 38.2052) ccw construction
  line L78 (-7.7948, 40.2052) -> (10.1151, 40.2052) construction
  line L79 (10.1151, 40.2052) -> (10.1151, 39.0783) construction
  arc A93 (9.7873, 38.6768) -> (10.1151, 39.0783) centre (9.7054, 39.0783) ccw construction
  arc A94 (9.7873, 38.6768) -> (10.2052, 34.5391) centre (10.2052, 36.6291) ccw construction
  line L80 (10.2052, 34.5391) -> (20.0038, 34.5391) construction
  arc A95 (20.0038, 34.5391) -> (20.5462, 38.647) centre (20.2052, 36.6023) ccw construction
  line L81 (20.5462, 38.647) -> (20.4256, 38.6775) construction
  arc A96 (20.0856, 39.0762) -> (20.4256, 38.6775) centre (20.4974, 39.083) ccw construction
  line L82 (0.2052, 32.2052) -> (30.2052, 32.2052) construction
  arc A97 (0.2052, 32.2052) -> (-1.7948, 30.2052) centre (0.2052, 30.2052) ccw construction
  line L83 (-1.7948, 30.2052) -> (-1.7948, 0.2052) construction
  arc A98 (-1.7948, 0.2052) -> (0.2052, -1.7948) centre (0.2052, 0.2052) ccw construction
  line L84 (0.2052, -1.7948) -> (30.2052, -1.7948) construction
  arc A99 (30.2052, -1.7948) -> (32.2052, 0.2052) centre (30.2052, 0.2052) ccw construction
  line L85 (32.2052, 0.2052) -> (32.2052, 30.2052) construction
  arc A100 (32.2052, 30.2052) -> (30.2052, 32.2052) centre (30.2052, 30.2052) ccw construction
  circle A101 centre (35.2052, 35.2052) radius 2.425 construction
  circle A102 centre (29.7052, 36.0052) radius 2.65 construction
  circle A103 centre (36.0052, 29.7052) radius 2.65 construction
  circle A104 centre (35.2052, -4.7948) radius 2.425 construction
  circle A105 centre (29.7052, -5.5948) radius 2.65 construction
  circle A106 centre (36.0052, 0.7052) radius 2.65 construction
  circle A107 centre (-4.7948, 35.2052) radius 2.425 construction
  circle A108 centre (0.7052, 36.0052) radius 2.65 construction
  circle A109 centre (-5.5948, 29.7052) radius 2.65 construction
  circle A110 centre (-5.5948, 0.7052) radius 2.65 construction
  circle A111 centre (0.7052, -5.5948) radius 2.65 construction
  circle A112 centre (-4.7948, -4.7948) radius 2.425 construction
  point P0 (0, 0)
  point P1 (-5.5744, -20.814)
hole "Hole2" at (5.5948, -49.2948, -5) at (-0.7052, -55.5948, -5) at (-29.7052, -55.5948, -5) at (-36.0052, -49.2948, -5) at (-36.0052, -20.2948, -5) at (-29.7052, -13.9948, -5) at (-0.7052, -13.9948, -5) at (5.5948, -20.2948, -5) at (5.5948, 0.7052, -5) at (-0.7052, -5.5948, -5) at (-29.7052, -5.5948, -5) at (-36.0052, 0.7052, -5) at (-36.0052, 29.7052, -5) at (-29.7052, 36.0052, -5) at (-0.7052, 36.0052, -5) at (5.5948, 29.7052, -5) direction (0, 0, 1) diameter 5 end through all
sketch "Sketch4" plane through (-38.2052, 40.2052, 0) normal (0, 1, 0) x (1, 0, 0)
  circle A0 centre (-6.3779, 23.8) radius 2.5
  circle A1 centre (-6.3779, 23.8) radius 4.55
  arc A2 (1.6221, 39.2) -> (1.6221, 43.4) centre (1.6221, 41.3) ccw
  circle A3 centre (1.6221, 6.3) radius 2.1
  line L0 (-0.8731, 5) -> (-2, 5)
  line L1 (-2, 5) -> (-2, 35)
  line L2 (-2, 35) -> (-2, 47.0302)
  line L3 (-2, 0) -> (-2, 5)
  line L4 (-2, 5) -> (-12, 5)
  line L5 (-12, 5) -> (-12, 47.0302)
  line L6 (-12, 47.0302) -> (-2, 47.0302)
  line L7 (-2, 47.0302) -> (-2, 5)
  circle A4 centre (-8.2796, 8.3) radius 2.1
  line L8 (-10.3779, 17.8) -> (-10.265, 17.8)
  line L9 (-10.3779, 51.8) -> (-6.4357, 51.8)
  line L10 (-10.3779, 17.8) -> (-10.3779, 51.8)
  arc A5 (-8.2796, 45.4) -> (-8.2796, 41.2) centre (-8.2796, 43.3) ccw
  circle A6 centre (-8.2796, 8.3) radius 1.45
  circle A7 centre (-8.2796, 43.3) radius 1.45
  line L11 (-2, 21.8) -> (18.1196, 21.8)
  line L12 (18.1196, 21.8) -> (18.1196, 5)
  line L13 (18.1196, 5) -> (-2, 5)
  line L14 (-2, 5) -> (-2, 21.8)
  line L15 (-12, 5) -> (0, 5)
  line L16 (0, 5) -> (0, 0)
  line L17 (0, 0) -> (-12, 0)
  line L18 (-12, 0) -> (-12, 5)
  line L19 (-10.265, 17.8) -> (-10.265, 51.2533)
  line L20 (-10.265, 51.2533) -> (-6.4357, 51.8)
  point P0 (38.2052, 0)
extrude "Extrusion2" add sketch "Sketch4" against normal blind 10 contours A0 | A1 L1 | L1 A1 L19 | A1 L19 L6 L2 L1 | L1 L4 L5 L6 L10 A1 L8 L19 | L19 A1 L10 | A1 L10 A5 L19 | L19 L8 L10 A1 | L11 L12 L13 A3 L0 L1 | L10 A1 | A5 L19 | L0 L13 A3 L16 L17 L3 | L3 L17 L18 L4 | L10 L6 L19 A5 | L13 L16 A3 | A3 L13 picked at (-0.003, 4.9812)
sketch "Sketch5" plane through (-38.2052, 30.2052, 0) normal (0, -1, 0) x (1, 0, 0)
  circle A0 centre (-6.3779, -23.8) radius 6 projected
  circle A1 centre (-16.2796, -25.8) radius 2.5 projected
  circle A2 centre (-16.2796, -25.8) radius 10.5309
  point P0 (38.2052, 0)
  constraints: 1 centre point
extrude "Extrusion3" cut sketch "Sketch5" against normal up to surface (10 mm away) contours A2 A0 | A0 A2 picked at (-8.2673, -22.7653) picked at (-14.5239, -19.9998)
body "Solid1"
